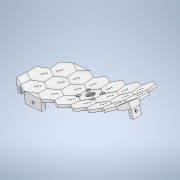
# Autodesk Inventor part: ArrayBracket
Saved by Autodesk Inventor 2022 (Build 260153070, 153G)
## iProperties
Created: 2021-11-12
Part Number: ArrayBracket
Material: PET Plastic
Document SubType Name: Modeling
Designer: elmar
Density: 1.541 g/cm^3
Appearance: White
Mass: 520.185 g
Surface Area: 474.933 cm^2
Volume: 337.563 cm^3
Author: elmar
Autodesk Inventor part; units mm, degrees
ref_plane "YZ Plane" through (0, 0, 0) normal (1, 0, 0) x (0, 1, 0)
ref_plane "XZ Plane" through (0, 0, 0) normal (0, 1, 0) x (-1, 0, 0)
ref_plane "XY Plane" through (0, 0, 0) normal (0, 0, 1) x (1, 0, 0)
sketch "Sketch1" plane through (0, 0, 0) normal (0, 0, 1) x (1, 0, 0)
  circle A0 centre (0, 0) radius 203
  line L0 (-129, -156.741826) -> (-129, -267)
  line L1 (-129, -267) -> (129, -267)
  line L2 (129, -267) -> (129, -156.741826)
  circle A1 centre (0, 0) radius 37
  line L3 (0, -203) -> (0, -267)
  line L4 (0, -235) -> (-129, -235)
  line L5 (0, -235) -> (11.5, -235)
  dimension "d0" = 406
  dimension "d1" = 267
  dimension "d2" = 74
  dimension "d3" = 258
  dimension "d11" = 11.5
  dimension "HalfAngle" = 2.802
  constraints: 12 end point, 3 perpendicular, 3 point on circle, 2 centre point, 2 coincident, 2 midpoint, 2 vertical, 1 horizontal, 1 parallel, 1 point on line
  measures "d0" diameter of A0
  measures "d1" distance from line of L1 point (0, 0)
  measures "d2" diameter of A1
  measures "d3" distance of L0.end L1.end
  measures "d11" distance of L4.start L5.end
extrude "Extrusion1" add sketch "Sketch1" along normal blind 74 contours A1
ref_plane "Work Plane1" through (0, -235, 0) normal (0, -1, 0) x (-1, 0, 0)
sketch "Sketch2" plane through (0, -235, 0) normal (0, -1, 0) x (-1, 0, 0)
  line L0 (0, 13.279056) -> (11.5, 6.639528)
  line L1 (11.5, 6.639528) -> (11.5, -6.639528)
  line L2 (11.5, -6.639528) -> (0, -13.279056)
  line L3 (0, -13.279056) -> (-11.5, -6.639528)
  line L4 (-11.5, -6.639528) -> (-11.5, 6.639528)
  line L5 (-11.5, 6.639528) -> (0, 13.279056)
  point P0 (0, 0)
  point P1 (0, 0)
  dimension "d8" = 23
  constraints: 12 end point, 1 coincident, 1 vertical, 13 other
  measures "d8" distance between parallel lines of L1 L4
extrude "Extrusion2" add sketch "Sketch2" along normal blind 3 draft 2.8016 separate body
sketch "Sketch3" plane through (0, -235, 0) normal (0, 1, 0) x (1, 0, 0)
  line L0 (-11.646809, -6.724288) -> (0, -13.448576)
  line L1 (0, 13.279056) -> (11.5, 6.639528)
  line L2 (0, 0) -> (5.75, 9.959292)
  point P0 (0.635, 1.099852)
  point P1 (1.905, 3.299557)
  point P2 (3.175, 5.499261)
  dimension "d16" = 1.27
  dimension "d17" = 2.54
  dimension "d18" = 2.54
  constraints: 3 point on line, 2 end point, 1 midpoint
  measures "d16" distance of L2.start point (0.635, 1.1)
  measures "d17" distance of point (0.635, 1.1) point (1.905, 3.3)
  measures "d18" distance of point (1.905, 3.3) point (3.175, 5.499)
hole "Hole1" at (1.905, -235, -3.299557) at (0.635, -235, -1.099852) at (3.175, -235, -5.499261) direction (0, -1, 0) diameter 1.27 end through all bodies 2
pattern_circular "Circular Pattern1" count 7 over 33.61921 about axis through (0, 0, -10) along (0, 0, 1) of "Extrusion2", "Hole1" bodies 2
ref_plane "Work Plane2" through (0, -235, -13.279056) normal (-0.0487035, 0.9952446, 0.0843569) x (0.8660254, 0, 0.5)
sketch "Sketch4" plane through (0, -235, -13.279056) normal (-0.0487035, 0.9952446, 0.0843569) x (0.8660254, 0, 0.5)
  line L0 (-0.047473, 22.972461) -> (13.215684, 22.999869)
  line L1 (13.215684, 22.999869) -> (19.870998, 11.527343)
  line L2 (19.870998, 11.527343) -> (13.263156, 0.027408)
  line L3 (13.263156, 0.027408) -> (0, 0)
  line L4 (0, 0) -> (-6.655315, 11.472526)
  line L5 (-6.655315, 11.472526) -> (-0.047473, 22.972461)
  point P0 (6.639528, 11.445313)
  point P1 (6.607842, 11.499935)
  point P2 (0, 0)
  constraints: 12 end point, 2 coincident, 13 other
extrude "Extrusion3" add sketch "Sketch4" against normal blind 3 draft 2.8016 separate body
sketch "Sketch5" plane through (0, -235, -13.279056) normal (-0.0487035, 0.9952446, 0.0843569) x (0.8660254, 0, 0.5)
  line L0 (6.639528, 11.445313) -> (6.639528, 10.175313)
  point P0 (6.639528, 7.635313)
  point P1 (6.639528, 5.095313)
  dimension "d29" = 2.54
  dimension "d30" = 2.54
  dimension "d199" = 1.27
  constraints: 3 end point, 2 point on line, 1 vertical
  measures "d29" distance of point (6.64, 7.635) L0.end
  measures "d30" distance of point (6.64, 5.095) point (6.64, 7.635)
  measures "d199" distance of L0.end L0.start
hole "Hole2" at (10.813463, -234.008854, -18.729467) at (9.549502, -234.256268, -16.540223) at (8.285542, -234.503681, -14.350979) direction (0.0487035, -0.9952446, -0.0843569) diameter 1.27 end through all bodies 3
pattern_circular "Circular Pattern2" count 6 over 28.01601 about axis through (0, 0, -10) along (0, 0, 1) of "Extrusion3" bodies 3
mirror "Mirror1" about plane through (0, 0, 0) normal (0, 0, 1) of "Extrusion3", "Circular Pattern2" bodies 3
ref_plane "Work Plane3" through (120.91255, -202.691008, -33.524907) normal (0, 0, 1) x (-0.957271, -0.2891923, 0)
sketch "Sketch16" plane through (79.062498, -221.604675, -6.696035) normal (0.2891923, -0.957271, 0) x (0.957271, 0.2891923, 0)
  line L0 (-1.437872, 0.346035) -> (-21.757872, 0.346035)
  line L1 (-21.757872, 0.346035) -> (-21.757872, 13.046035)
  line L2 (-21.757872, 13.046035) -> (-1.437872, 13.046035)
  line L3 (-1.437872, 13.046035) -> (-1.437872, 0.346035)
  line L4 (-1.437872, 0.346035) -> (-21.757872, 13.046035) construction
  line L5 (-21.757872, 0.346035) -> (-1.437872, 13.046035) construction
  circle A0 centre (-21.757872, 13.046035) radius 1.2
  circle A1 centre (-1.437872, 13.046035) radius 1.2
  circle A2 centre (-21.757872, 0.346035) radius 1.2
  circle A3 centre (-1.437872, 0.346035) radius 1.2
  circle A4 centre (-10.962872, 5.596182) radius 0.635
  circle A5 centre (-8.422872, 1.196773) radius 0.635
  circle A6 centre (-9.692872, 3.396478) radius 0.635
  line L6 (0.048936, -0.028253) -> (-11.597872, -6.752541)
  line L7 (0.048936, 13.420323) -> (0.048936, -0.028253)
  line L8 (-11.597872, 20.144611) -> (0.048936, 13.420323)
  line L9 (-23.244681, 13.420323) -> (-11.597872, 20.144611)
  line L10 (-23.244681, 13.420323) -> (-23.244681, -0.028253)
  line L11 (-11.597872, -6.752541) -> (-23.244681, -0.028253)
  point P0 (-11.597872, 6.696035)
  dimension "d94" = 12.7
  dimension "d95" = 20.32
  dimension "d96" = 2.4
  constraints: 12 end point, 8 coincident, 4 centre point, 3 equal radius, 2 midpoint, 2 parallel, 1 horizontal, 1 perpendicular
  measures "d94" distance of L0.end L1.end
  measures "d95" distance of L1.end L2.end
  measures "d96" diameter of A0
extrude "Extrusion11" add sketch "Sketch16" along normal up to surface (3 mm away) contours A2 L11 L1 L0 | A2 L1 A0 L2 A1 L3 A3 L0 | L0 L1 A2 | L0 A3 L6 L11 A2 | A3 L3 L0 | L0 L3 A3 L6 | A2 L11 L10 L9 A0 L1 | L3 A1 L8 L7 L6 A3 | A0 L9 L2 L1 | L1 L2 A0 | A1 L2 L3 | L3 L2 A1 L8 | A0 L9 L8 A1 L2 | A4 | A5 | A6 bodies 2
extrude "Extrusion10" [suppressed]
hole "Hole5" at (67.960191, -224.958691, 0) direction (0.2891923, -0.957271, 0) diameter 10 end through all bodies 2
ref_plane "Work Plane9" through (67.635469, -223.883813, 26.526539) normal (0.957271, 0.2891923, 0) x (0.2873565, -0.9511941, 0.1124989)
hole "Hole9" at (58.234317, -227.896884, -6.35) at (58.234317, -227.896884, 6.35) at (77.686064, -222.020497, 6.35) at (77.686064, -222.020497, -6.35) direction (0.2891923, -0.957271, 0) diameter 2.9 end through all countersink diameter 5.5 countersink angle 90 bodies 2 3 clearance for "Flat Head Machine Screw" size "M2.5" standard "Ansi Metric M Profile"
sketch "Sketch20" plane through (78.968807, -221.632979, 3.948563) normal (-0.2891923, 0.957271, 0) x (0.957271, 0.2891923, 0)
  arc A0 (-24.222288, 11.297151) -> (-23, 7.897126) centre (-21.66, 10.298563) ccw
  arc A1 (-19.892485, 12.405312) -> (-24.2132, 11.320165) centre (-21.66, 10.298563) ccw
  arc A2 (-23, 7.897126) -> (-19.998977, 12.490252) centre (-21.66, 10.298563) ccw
  arc A3 (-19.998977, -4.593126) -> (-23, 0) centre (-21.66, -2.401437) ccw
  arc A4 (-23, 0) -> (-24.222288, -3.400025) centre (-21.66, -2.401437) ccw
  arc A5 (-24.2132, -3.423039) -> (-19.892485, -4.508186) centre (-21.66, -2.401437) ccw
  arc A6 (0, 0) -> (-3.001023, -4.593126) centre (-1.34, -2.401437) ccw
  arc A7 (-3.001023, 12.490252) -> (0, 7.897126) centre (-1.34, 10.298563) ccw
  circle A8 centre (-21.66, -2.401437) radius 2.75
  circle A9 centre (-21.66, 10.298563) radius 2.75
  circle A10 centre (-1.34, -2.401437) radius 2.75
  line L0 (0, 10.588091) -> (0, 0)
  circle A11 centre (-1.34, 10.298563) radius 2.75
  point P0 (-11.5, 3.948563)
  point P1 (-3.001023, 12.490252)
  point P2 (0, 0)
  point P3 (-24.2132, -3.423039)
  point P4 (-23.071688, 11.286294)
  point P5 (-23, 10.401194)
  point P6 (-21.178594, 12.322932)
  point P7 (-23.06494, 11.313848)
  point P8 (-23, -1.190835)
  point P9 (-23.071688, -2.075936)
  point P10 (-23.06494, -2.10349)
  point P11 (-21.178594, -3.112574)
  point P12 (0, 10.401194)
  point P13 (-19.998977, 12.490252)
  point P14 (-23, 7.897126)
  point P15 (-23, 0)
  point P16 (-19.998977, -4.593126)
  constraints: 4 coincident, 12 other
extrude "Extrusion14" cut sketch "Sketch20" along normal through all bodies 2 3
ref_plane "Work Plane12" through (-11.5, -235, 6.639528) normal (0.0484735, 0.9952895, -0.0839586) x (0.4988107, 0.0487031, 0.8653415)
ref_plane "Work Plane13" through (0, -238, -13.448576) normal (-0.2891923, 0.957271, 0) x (0.957271, 0.2891923, 0)
sketch "Sketch27" plane through (-11.5, -235, 6.639528) normal (0.0484735, 0.9952895, -0.0839586) x (0.4988107, 0.0487031, 0.8653415)
  line L0 (0, 0) -> (-11.490918, 6.561185)
  line L1 (22.945205, 0) -> (11.481782, 6.670983)
  line L2 (11.481782, 6.670983) -> (0, 0)
  line L3 (22.945205, 0) -> (11.481782, 6.670983)
  line L4 (11.481782, 6.670983) -> (0, 0)
  line L5 (0, 0) -> (11.463423, -6.670983)
  line L6 (11.463423, -6.670983) -> (22.945205, 0)
  point P0 (11.436101, -6.466837)
  constraints: 8 end point, 3 equal length
extrude "Extrusion19" add sketch "Sketch27" against normal up to surface surface through (0, -238, -13.448576) normal (-0.2891923, 0.957271, 0) bodies 2
sketch "Sketch28" plane through (-11.820019, -241.570837, 7.193817) normal (0.2891923, -0.957271, 0) x (0.8492534, 0.2565601, 0.4614602)
  line L0 (0.925735, 2.030425) -> (6.040789, 11.864157)
  line L1 (6.040789, 11.864157) -> (9.944297, 9.833732)
  line L2 (9.944297, 9.833732) -> (4.829243, 0)
  line L3 (4.829243, 0) -> (0.925735, 2.030425)
  line L4 (-69.79898, 28.197405) -> (243.023514, -134.518439)
  line L5 (8.04069, 10.089671) -> (6.040789, 11.864157)
  line L6 (0, 0) -> (13.743516, 0)
  point P0 (68.69597, -43.841285)
  dimension "d167" = 4.4
  constraints: 8 end point, 3 parallel, 1 perpendicular, 1 point on line
  measures "d167" distance of L2.end L0.start
extrude "Extrusion20" add sketch "Sketch28" along normal up to surface (10.169496 mm away) bodies 2
sketch "Sketch29" plane through (-7.718768, -240.331846, 20.506817) normal (0.957271, 0.2891923, 0) x (0, 0, -1)
  line L0 (7.129961, -1) -> (8.717675, -3.75)
  line L1 (8.717675, -3.75) -> (7.129961, -6.5)
  line L2 (7.129961, -6.5) -> (3.954535, -6.5)
  line L3 (3.954535, -6.5) -> (2.366822, -3.75)
  line L4 (2.366822, -3.75) -> (3.954535, -1)
  line L5 (3.954535, -1) -> (7.129961, -1)
  line L6 (0, 0) -> (11.084496, 0)
  line L7 (5.542248, 0) -> (5.542248, -10.169496)
  line L8 (0, -10.169496) -> (11.084496, -10.169496)
  point P0 (20.506817, 227.830504)
  point P1 (5.542248, -3.75)
  point P2 (5.542248, -3.75)
  dimension "d170" = 5.5
  dimension "d195" = 1
  constraints: 14 end point, 2 midpoint, 1 coincident, 1 point on line, 13 other
  measures "d170" distance between parallel lines of L3 L0
  measures "d195" distance between parallel lines of L5 L6
extrude "Extrusion21" cut sketch "Sketch29" against normal blind 2.4 bodies 2
hole "Hole11" at (-6.634297, -243.921612, 14.964569) direction (-0.957271, -0.2891923, 0) diameter 3.4 end through all bodies 2 clearance for "Flat Head Machine Screw" size "M3" standard "Ansi Metric M Profile"
mirror "Mirror6" about plane through (67.635469, -223.883813, 26.526539) normal (0.957271, 0.2891923, 0) of "Extrusion20", "Extrusion21", "Hole11", "Extrusion19" bodies 2
sketch "Sketch30" plane through (11.499869, -234.99733, 6.671101) normal (-0.0487035, 0.9952446, -0.0843569) x (0.8629287, 0.0844573, 0.4982178)
  line L0 (6.600019, -11.431568) -> (6.623671, 0.013721)
  line L1 (13.263185, 0) -> (-0.015843, 0.027441)
  point P0 (6.602644, -10.161568)
  point P1 (6.607892, -7.621568)
  point P2 (6.613141, -5.081568)
  dimension "d183" = 1.27
  dimension "d185" = 2.54
  dimension "d186" = 2.54
  constraints: 3 point on line, 2 end point, 1 midpoint
  measures "d183" distance of L0.start point (6.603, -10.162)
  measures "d185" distance of point (6.608, -7.622) point (6.603, -10.162)
  measures "d186" distance of point (6.608, -7.622) point (6.613, -5.082)
hole "Hole12" at (12.086484, -233.946557, 18.729465) at (13.368565, -234.069378, 16.540216) at (14.650647, -234.192198, 14.350967) direction (0.0487035, -0.9952446, 0.0843569) diameter 1.27 end through all bodies 3
pattern_circular "Circular Pattern4" count 6 over 28.01601 about axis through (0, 0, -10) along (0, 0, 1) of "Hole2", "Hole12" bodies 3
ref_plane "Work Plane14" through (23.126936, -235.731083, 26.864571) normal (-0.0976385, 0.9952219, 0) x (0.9952219, 0.0976385, 0)
ref_plane "Work Plane15" through (22.890366, -232.759654, 26.494966) normal (0.0962651, -0.9812233, 0.1671345) x (-0.8670519, -0.0002013, 0.4982178)
sketch "Sketch31" plane through (23.126936, -235.731083, 26.864571) normal (-0.0976385, 0.9952219, 0) x (0.9952219, 0.0976385, 0)
  line L0 (0, 0.338032) -> (-11.390497, -6.238349)
  line L1 (11.390497, -6.238349) -> (0, 0.338032)
  line L2 (11.390497, -6.238349) -> (11.535908, -6.660335)
  line L3 (-11.390497, -6.238349) -> (11.390497, -6.238349)
  constraints: 2 end point, 1 horizontal
extrude "Extrusion22" add sketch "Sketch31" along normal up to surface surface through (22.890366, -232.759654, 26.494966) normal (0.0962651, -0.9812233, 0.1671345) bodies 2
sketch "Sketch32" plane through (23.126936, -235.731083, 26.864571) normal (0.0976385, -0.9952219, 0) x (0.9952219, 0.0976385, 0)
  line L0 (-11.390497, 6.238349) -> (11.390497, 6.238349)
  line L1 (11.390497, 6.238349) -> (11.390497, 0.838349)
  line L2 (11.390497, 0.838349) -> (-11.390497, 0.838349)
  line L3 (-11.390497, 0.838349) -> (-11.390497, 6.238349)
  line L4 (-11.390497, 6.238349) -> (11.390497, 0.838349) construction
  line L5 (11.390497, 6.238349) -> (-11.390497, 0.838349) construction
  point P0 (0, -26.864571)
  point P1 (0, 3.538349)
  dimension "d198" = 5.4
  constraints: 12 end point, 2 coincident, 2 midpoint, 2 parallel, 1 horizontal, 1 perpendicular
  measures "d198" distance of L0.end L1.end
extrude "Extrusion23" add sketch "Sketch32" along normal blind 10 and the other way blind 2 bodies 2
sketch "Sketch33" plane through (25.154729, -235.532142, 27.70292) normal (0, 0, -1) x (-0.9952219, -0.0976385, 0)
  line L0 (13.428025, -10) -> (-9.352968, -10)
  line L1 (2.037529, -1.137224) -> (-9.60915, -1.13452)
  line L2 (5.213128, -4.287207) -> (3.625415, -7.037207)
  line L3 (3.625415, -7.037207) -> (0.449989, -7.037207)
  line L4 (0.449989, -7.037207) -> (-1.137724, -4.287207)
  line L5 (-1.137724, -4.287207) -> (0.449989, -1.537207)
  line L6 (0.449989, -1.537207) -> (3.625415, -1.537207)
  line L7 (3.625415, -1.537207) -> (5.213128, -4.287207)
  line L8 (2.093086, -0.000052) -> (2.037702, -1.137207)
  line L9 (2.037702, -1.137207) -> (2.037702, -1.537207)
  point P0 (2.037529, 236.862827)
  point P1 (2.037702, -4.287207)
  dimension "d205" = 5.5
  dimension "d206" = 0.4
  constraints: 14 end point, 1 midpoint, 1 parallel, 1 perpendicular, 13 other
  measures "d205" distance between parallel lines of L3 L6
  measures "d206" distance of L8.end L9.end
extrude "Extrusion24" cut sketch "Sketch33" against normal blind 2.4 bodies 2
hole "Hole13" at (23.54536, -239.997823, 27.70292) direction (0, 0, 1) diameter 3.4 end through all bodies 2 clearance for "Flat Head Machine Screw" size "M3" standard "Ansi Metric M Profile"
mirror "Mirror7" about plane through (0, 0, 0) normal (0, 0, 1) of "Extrusion23", "Extrusion24", "Hole13", "Extrusion22" bodies 2
equation "\"d11\" = 0.5 * d8"
equation "\"d10\" = HalfAngle"
equation "\"d14\" = 12 * HalfAngle"
equation "\"d27\" = HalfAngle"
equation "\"d39\" = 10 * HalfAngle"
equation "\"d181\" = 10 * HalfAngle"
body "Solid1"
body "Solid2"
body "Solid3"
